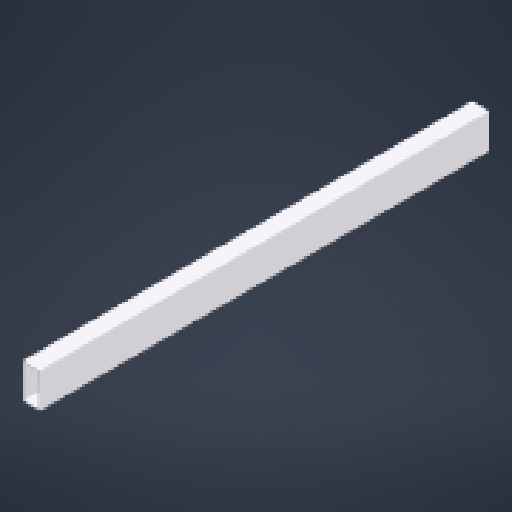
# Autodesk Inventor part: CRASH_BAR_INTAKE
Saved by Autodesk Inventor 2026.2 (Build 302298010, 298A)
## iProperties
Created: 2026-04-01
Part Number: CRASH_BAR_INTAKE
Material: Aluminum, 6061-T6
Document SubType Name: Modeling
Designer: 4aida
Density: 2.71 g/cm^3
Appearance: Metal-AL-6061 (Flat)
Author: 4aida
Autodesk Inventor part; units mm, degrees
ref_plane "YZ Plane" through (0, 0, 0) normal (1, 0, 0) x (0, 1, 0)
ref_plane "XZ Plane" through (0, 0, 0) normal (0, 1, 0) x (-1, 0, 0)
ref_plane "XY Plane" through (0, 0, 0) normal (0, 0, 1) x (1, 0, 0)
sketch "Sketch1" plane through (0, 0, 0) normal (0, 0, 1) x (1, 0, 0)
  line L0 (12.7, -25.4) -> (-12.7, -25.4)
  line L1 (-12.7, -25.4) -> (-12.7, 25.4)
  line L2 (-12.7, 25.4) -> (12.7, 25.4)
  line L3 (12.7, 25.4) -> (12.7, -25.4)
  line L4 (12.7, -25.4) -> (-12.7, 25.4) construction
  line L5 (-12.7, -25.4) -> (12.7, 25.4) construction
  line L6 (11.1125, -23.8125) -> (-11.1125, -23.8125)
  line L7 (-11.1125, -23.8125) -> (-11.1125, 23.8125)
  line L8 (-11.1125, 23.8125) -> (11.1125, 23.8125)
  line L9 (11.1125, 23.8125) -> (11.1125, -23.8125)
  line L10 (11.1125, -23.8125) -> (-11.1125, 23.8125) construction
  line L11 (-11.1125, -23.8125) -> (11.1125, 23.8125) construction
  point P0 (0, 0)
  dimension "d0" = 1.5875
  dimension "d1" = 1.5875
  dimension "d2" = 25.4
  dimension "d3" = 50.8
  constraints: 24 end point, 4 midpoint, 4 parallel, 2 horizontal, 2 perpendicular
  measures "d0" distance between parallel lines of L2 L8
  measures "d1" distance between parallel lines of L7 L1
  measures "d2" distance of L1.end L2.end
  measures "d3" distance of L0.end L1.end
extrude "Extrusion1" add sketch "Sketch1" along normal mid plane 631.698
sketch "Sketch2" plane through (12.7, -25.4, 315.849) normal (1, 0, 0) x (0, 0, -1)
  line L0 (0, 0) -> (0, 50.8) projected
  point P0 (315.849, 25.4)
  point P1 (5, 25.4)
  point P2 (17, 25.4)
  point P3 (0, 25.4)
  dimension "d6" = 12
  dimension "d7" = 5
  constraints: 2 horizontal alignment, 1 midpoint
  measures "d6" distance of point (5, 25.4) point (17, 25.4)
  measures "d7" distance from line of L0 point (5, 25.4)
hole "Hole1" at (12.7, 0, 310.849) at (12.7, 0, 298.849) direction (-1, 0, 0) diameter 5.105 end through all clearance for "Flat Head Machine Screw (82)" size "#10" standard "Ansi Unified Screw Threads"
mirror "Mirror1" about plane through (0, 0, 0) normal (0, 0, 1) of "Hole1"
sketch "Sketch3" plane through (12.7, -25.4, 315.849) normal (1, 0, 0) x (0, 0, -1)
  line L0 (631.698, 0) -> (0, 0) projected
  point P0 (315.849, 25.4)
  point P1 (315.849, 25.4)
  point P2 (265.049, 25.4)
  point P3 (214.249, 25.4)
  point P4 (163.449, 25.4)
  point P5 (112.649, 25.4)
  point P6 (61.849, 25.4)
  point P7 (366.649, 25.4)
  point P8 (315.849, 25.4)
  point P9 (265.049, 25.4)
  point P10 (214.249, 25.4)
  point P11 (163.449, 25.4)
  point P12 (112.649, 25.4)
  point P13 (417.449, 25.4)
  point P14 (366.649, 25.4)
  point P15 (315.849, 25.4)
  point P16 (265.049, 25.4)
  point P17 (214.249, 25.4)
  point P18 (163.449, 25.4)
  point P19 (468.249, 25.4)
  point P20 (417.449, 25.4)
  point P21 (366.649, 25.4)
  point P22 (315.849, 25.4)
  point P23 (265.049, 25.4)
  point P24 (214.249, 25.4)
  point P25 (519.049, 25.4)
  point P26 (468.249, 25.4)
  point P27 (417.449, 25.4)
  point P28 (366.649, 25.4)
  point P29 (315.849, 25.4)
  point P30 (265.049, 25.4)
  point P31 (569.849, 25.4)
  point P32 (519.049, 25.4)
  point P33 (468.249, 25.4)
  point P34 (417.449, 25.4)
  point P35 (366.649, 25.4)
  point P36 (315.849, 25.4)
  dimension "d17" = 50.8
  dimension "d20" = 50.8
  constraints: 2 horizontal, 1 coincident, 35 other
  measures "d17" distance of point (315.849, 25.4) point (265.049, 25.4)
  measures "d20" distance of point (315.849, 25.4) point (366.649, 25.4)
hole "Hole2" at (12.7, 0, 0) at (12.7, 0, 50.8) at (12.7, 0, 101.6) at (12.7, 0, 152.4) at (12.7, 0, 203.2) at (12.7, 0, 254) at (12.7, 0, -50.8) at (12.7, 0, -101.6) at (12.7, 0, -152.4) at (12.7, 0, -203.2) at (12.7, 0, -254) direction (-1, 0, 0) diameter 5.105 end through all clearance for "Flat Head Machine Screw (82)" size "#10" standard "Ansi Unified Screw Threads"
equation "\"d1\" = d0"
body "Solid1"
